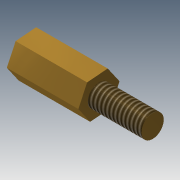
# Autodesk Inventor part: standoff
Saved by Autodesk Inventor 2014 SP1 (Build 180222100, 222)
## iProperties
Created: 2014-08-13
Part Number: standoff
Material: Brass, Soft Yellow
Document SubType Name: Modeling
Designer: James
Density: 8.47 g/cm^3
Appearance: Brass - Satin
Author: James
Autodesk Inventor part; units mm, degrees
ref_plane "YZ Plane" through (0, 0, 0) normal (1, 0, 0) x (0, 1, 0)
ref_plane "XZ Plane" through (0, 0, 0) normal (0, 1, 0) x (-1, 0, 0)
ref_plane "XY Plane" through (0, 0, 0) normal (0, 0, 1) x (1, 0, 0)
sketch "Sketch1" plane through (0, 0, 0) normal (1, 0, 0) x (0, 1, 0)
  line L0 (-10.311, 3.6207) -> (-11.2914, 1.5298)
  line L1 (-11.2914, 1.5298) -> (-13.5924, 1.3333)
  line L2 (-13.5924, 1.3333) -> (-14.913, 3.2279)
  line L3 (-14.913, 3.2279) -> (-13.9326, 5.3188)
  line L4 (-13.9326, 5.3188) -> (-11.6316, 5.5153)
  line L5 (-11.6316, 5.5153) -> (-10.311, 3.6207)
  point P0 (0, 0)
  point P1 (-12.612, 3.4243)
  dimension "d0" = 2
  constraints: 12 end point, 13 other
  measures "d0" distance from line of point (-12.612, 3.424) L5
extrude "Extrusion1" add sketch "Sketch1" along normal blind 8
sketch "Sketch2" plane through (8, 0, 0) normal (1, 0, 0) x (0, 0, -1)
  line L0 (-3.6207, -10.311) -> (-5.5153, -11.6316) projected
  line L1 (-3.2279, -14.913) -> (-1.3333, -13.5924) projected
  line L2 (-4.568, -10.9713) -> (-2.2806, -14.2527)
  circle A0 centre (-3.4243, -12.612) radius 1.25
  point P0 (0, 0)
  dimension "d3" = 2.5
  constraints: 3 midpoint, 2 end point, 1 centre point, 1 coincident
  measures "d3" diameter of A0
extrude "Extrusion2" add sketch "Sketch2" along normal blind 6
thread "Thread1" size "M2.5x0.45" class "6g" standard "ANSI Metric M Profile" full length
sketch "Sketch3" plane through (0, 0, 0) normal (-1, 0, 0) x (0, 0, 1)
  line L0 (1.3333, -13.5924) -> (3.2279, -14.913) projected
  line L1 (5.5153, -11.6316) -> (3.6207, -10.311) projected
  line L2 (4.568, -10.9713) -> (2.2806, -14.2527)
  point P0 (0, 0)
  point P1 (3.4243, -12.612)
  constraints: 3 midpoint, 2 end point
hole "Hole1" at (0, -12.612, 3.4243) direction (1, 0, 0) diameter 2.013 depth 5 tip angle 118 thread size "M2.5x0.45" class "6H" standard "ANSI Metric M Profile"
body "Solid1"
